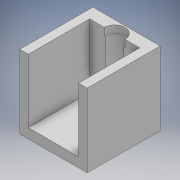
# Autodesk Inventor part: mini_holder
Saved by Autodesk Inventor 2017 (Build 210142000, 142)
## iProperties
Part Number: mini_holder
Material: Типовые
Document SubType Name: Modeling
Designer: Tolya
Density: 1 g/cm^3
Appearance: По умолчанию
Author: Tolya
Autodesk Inventor part; units mm, degrees
ref_plane "YZ Plane" through (0, 0, 0) normal (1, 0, 0) x (0, 1, 0)
ref_plane "XZ Plane" through (0, 0, 0) normal (0, 1, 0) x (-1, 0, 0)
ref_plane "XY Plane" through (0, 0, 0) normal (0, 0, 1) x (1, 0, 0)
sketch "Эскиз1" plane through (0, 0, 0) normal (0, 0, 1) x (1, 0, 0)
  arc A0 (3.75, 0) -> (-3.75, 0) centre (0, 0) ccw
  line L0 (-3.75, 0) -> (-13.75, 0) construction
  line L1 (-13.75, 4.8279) -> (13.75, 4.8279)
  line L2 (-13.75, 0) -> (-3.75, 0)
  line L3 (3.75, 0) -> (13.75, 0)
  line L4 (0, 9.2451) -> (0, -5.452)
  line L5 (-13.75, 0) -> (-13.75, 4.8279)
  line L6 (13.75, 0) -> (13.75, 4.8279)
  point P0 (0, 4.8279)
  dimension "d25" = 3.75
  constraints: 14 end point, 2 horizontal, 2 point on circle, 2 symmetric about line, 1 centre point, 1 collinear, 1 midpoint, 1 perpendicular, 1 point on line, 1 vertical
  measures "d25" radius of A0
extrude "Выдавливание1" add sketch "Эскиз1" along normal blind 30
sketch "Эскиз4" plane through (0, 0, 30) normal (0, 0, 1) x (1, 0, 0)
  circle A0 centre (0, 0) radius 4.25
  dimension "d22" = 8.5
  constraints: 1 centre point, 1 coincident
  measures "d22" diameter of A0
extrude "Выдавливание4" cut sketch "Эскиз4" against normal blind 3
sketch "Эскиз5" plane through (-13.75, 0, 0) normal (0, -1, 0) x (1, 0, 0)
  line L0 (23.75, -2.1369) -> (23.75, 32.4902)
  line L1 (27.5, 30) -> (0, 30) projected
  line L2 (0, 30) -> (3.5, 30)
  line L3 (0, 30) -> (0, 0)
  line L4 (0, 0) -> (27.5, 0) projected
  line L5 (0, 0) -> (27.5, 0)
  line L6 (27.5, 0) -> (27.5, 30)
  line L7 (27.5, 30) -> (24, 30)
  line L8 (3.5, 4) -> (24, 4)
  line L9 (24, 4) -> (24, 30)
  line L10 (3.5, 30) -> (3.5, 4)
  point P0 (13.75, 0)
  dimension "d26" = 3.5
  dimension "d27" = 3.5
  constraints: 18 end point, 4 perpendicular, 2 point on line, 2 vertical, 1 horizontal
  measures "d26" distance of L1.end L2.end
  measures "d27" distance of L1.start L7.end
extrude "Выдавливание5" add sketch "Эскиз5" along normal blind 25 contours L4 L3 L1 L10 L8 L0 | L0 L8 L9 L1 L6 L4
sketch "Эскиз6" plane through (-3.75, 0, 4) normal (0, 0, 1) x (1, 0, 0)
  circle A0 centre (3.75, 0) radius 3.75
  constraints: 1 centre point, 1 coincident
extrude "Выдавливание6" cut sketch "Эскиз6" against normal blind 25
